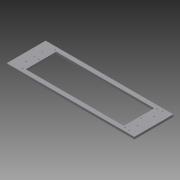
# Autodesk Inventor part: core xy gantry
Saved by Autodesk Inventor 2014 SP1 (Build 180222100, 222)
## iProperties
Created: 2014-09-21
Part Number: core xy gantry
Material: Generic
Document SubType Name: Modeling
Designer: Mon
Density: 1 g/cm^3
Appearance: Default
Author: Mon
Autodesk Inventor part; units mm, degrees
ref_plane "YZ Plane" through (0, 0, 0) normal (1, 0, 0) x (0, 1, 0)
ref_plane "XZ Plane" through (0, 0, 0) normal (0, 1, 0) x (-1, 0, 0)
ref_plane "XY Plane" through (0, 0, 0) normal (0, 0, 1) x (1, 0, 0)
sketch "Sketch1" plane through (0, 0, 0) normal (0, 1, 0) x (-1, 0, 0)
  line L0 (283.4202, -0.0606) -> (0.0202, -0.0606)
  circle A0 centre (28.4702, 43.2144) radius 1
  circle A1 centre (28.4702, 79.0269) radius 1
  circle A2 centre (28.4702, 7.4019) radius 1
  circle A3 centre (254.9702, 7.4019) radius 1
  circle A4 centre (254.9702, 43.2144) radius 1
  circle A5 centre (254.9702, 79.0269) radius 1
  circle A6 centre (17.6702, 6.2894) radius 1
  circle A7 centre (17.6702, 80.1394) radius 1
  circle A8 centre (265.7702, 43.2144) radius 1
  line L1 (283.4202, 86.4894) -> (283.4202, -0.0606)
  line L2 (250.4702, 76.9644) -> (250.4702, 9.4644)
  line L3 (32.9702, 76.9644) -> (250.4702, 76.9644)
  line L4 (32.9702, 9.4644) -> (32.9702, 76.9644)
  line L5 (250.4702, 9.4644) -> (32.9702, 9.4644)
  line L6 (0.0202, -0.0606) -> (0.0202, 86.4894)
  line L7 (0.0202, 86.4894) -> (283.4202, 86.4894)
  circle A9 centre (17.9702, 24.9144) radius 1
  circle A10 centre (265.4702, 24.9144) radius 1
  circle A11 centre (265.4702, 61.5144) radius 1
  circle A12 centre (17.9702, 61.5144) radius 1
  point P0 (0, 0)
  constraints: 16 end point, 13 centre point
extrude "Extrusion1" add sketch "Sketch1" along normal blind 4.7625
body "Solid1"
